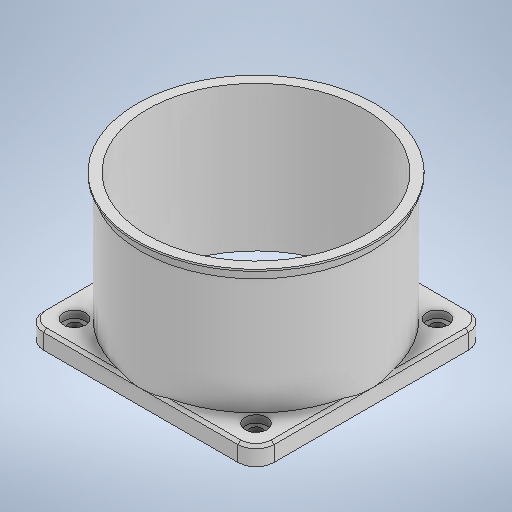
# Autodesk Inventor part: fanHoseMount
Saved by Autodesk Inventor 2025.1 (Build 291241000, 241)
## iProperties
Created: 2024-09-02
Part Number: fanHoseMount
Material: Generic
Document SubType Name: Modeling
Designer: Eric
Density: 1 g/cm^3
Appearance: Default
Author: Eric
Autodesk Inventor part; units mm, degrees
ref_plane "YZ Plane" through (0, 0, 0) normal (1, 0, 0) x (0, 1, 0)
ref_plane "XZ Plane" through (0, 0, 0) normal (0, 1, 0) x (-1, 0, 0)
ref_plane "XY Plane" through (0, 0, 0) normal (0, 0, 1) x (1, 0, 0)
sketch "Sketch1" plane through (0, 0, 0) normal (0, 1, 0) x (-1, 0, 0)
  circle A0 centre (0, 0) radius 30
  line L0 (26.75, -31.75) -> (-26.75, -31.75)
  line L1 (-31.75, -26.75) -> (-31.75, 26.75)
  line L2 (-26.75, 31.75) -> (26.75, 31.75)
  line L3 (31.75, 26.75) -> (31.75, -26.75)
  circle A1 centre (25, -25) radius 1.75
  circle A2 centre (-25, -25) radius 1.75
  circle A3 centre (-25, 25) radius 1.75
  circle A4 centre (25, 25) radius 1.75
  arc A5 (26.75, -31.75) -> (31.75, -26.75) centre (26.75, -26.75) ccw
  arc A6 (31.75, 26.75) -> (26.75, 31.75) centre (26.75, 26.75) ccw
  arc A7 (-26.75, 31.75) -> (-31.75, 26.75) centre (-26.75, 26.75) ccw
  arc A8 (-31.75, -26.75) -> (-26.75, -31.75) centre (-26.75, -26.75) ccw
  point P0 (31.75, -31.75)
  point P1 (0, -31.75)
  point P2 (-31.75, 0)
  dimension "d1" = 3.5
  dimension "d2" = 60
  dimension "d3" = 50
  dimension "d4" = 50
  dimension "d5" = 25
  dimension "d6" = 25
  dimension "d7" = 5
  dimension "d8" = 5
  dimension "d9" = 63.5
  dimension "d10" = 63.5
  constraints: 9 centre point, 8 end point, 8 point on circle, 8 tangent, 5 equal radius, 3 horizontal alignment, 3 vertical alignment, 2 midpoint, 2 parallel, 2 point on line, 1 coincident, 1 horizontal, 1 perpendicular
  measures "d1" diameter of A2
  measures "d2" diameter of A0
  measures "d3" distance of A1.centre A2.centre
  measures "d4" distance of A2.centre A3.centre
  measures "d5" horizontal distance of point (0, 0) A2.centre
  measures "d6" horizontal distance of point (0, 0) A2.centre
  measures "d7" radius of A5
  measures "d8" radius of A6
  measures "d9" distance between parallel lines of L2 L0
  measures "d10" distance between parallel lines of L3 L1
extrude "Extrusion1" add sketch "Sketch1" along normal blind 5
sketch "Sketch2" plane through (0, 5, 0) normal (0, 1, 0) x (1, 0, 0)
  circle A0 centre (-25, -25) radius 1.75 projected
  circle A1 centre (-25, -25) radius 3
  circle A2 centre (-25, 25) radius 1.75 projected
  circle A3 centre (-25, 25) radius 3
  circle A4 centre (25, 25) radius 1.75 projected
  circle A5 centre (25, 25) radius 3
  circle A6 centre (25, -25) radius 1.75 projected
  circle A7 centre (25, -25) radius 3
  point P0 (0, 0)
  dimension "d13" = 6
  constraints: 4 centre point, 4 coincident, 3 equal radius
  measures "d13" diameter of A1
extrude "Extrusion2" cut sketch "Sketch2" against normal blind 2 contours A0 | A1 | A2 | A3 | A4 | A5 | A6 | A7
sketch "Sketch3" plane through (0, 0, 0) normal (0, 0, 1) x (1, 0, 0)
  line L0 (-26.75, 5) -> (26.75, 5) projected
  line L1 (0, 5) -> (0, 15)
  arc A0 (0, 15) -> (0, 15) centre (30, 15) ccw
  line L2 (0, 15) -> (0, 40)
  point P0 (0, 0)
  dimension "d16" = 180
  dimension "d17" = 30
  dimension "d18" = 25
  dimension "d19" = 10
  constraints: 4 end point, 2 point on circle, 2 tangent, 1 centre point, 1 midpoint, 1 vertical
  measures "d16" angle of L1 L2
  measures "d17" radius of A0
  measures "d18" distance of L2.start L2.end
  measures "d19" distance of L1.start L1.end
sketch "Sketch4" plane through (0, 5, 0) normal (0, 1, 0) x (1, 0, 0)
  circle A0 centre (0, 0) radius 31.75
  line L0 (26.75, 31.75) -> (-26.75, 31.75) projected
  circle A1 centre (0, 0) radius 30 projected
  constraints: 1 centre point, 1 coincident, 1 tangent
sweep "Sweep1" add profiles "Sketch4" path "Sketch3" path curves L1 L2
sketch "Sketch5" plane through (0, 40, 0) normal (0, 1, 0) x (0, 0, -1)
  circle A0 centre (0, 0) radius 31.75 projected
  circle A1 centre (0, 0) radius 32.75
  point P0 (0, 0)
  dimension "d22" = 1
  constraints: 1 centre point
  measures "d22" radial gap between concentric circles of A0 A1
extrude "Extrusion3" add sketch "Sketch5" against normal blind 3
chamfer "Chamfer1" distance 1 distance2 2.5 1 edges at (0, 37, 32.75) measured on face at (0, 37, 32.25)
chamfer "Chamfer2" distance 0.75 angle 45 12 edges at (-31.75, 5, -13.375) (-30.2855, 5, -30.2855) (-13.375, 5, -31.75) (-31.75, 5, 13.375) (-30.2855, 5, 30.2855) (-13.375, 5, 31.75) (13.375, 5, -31.75) (30.2855, 5, -30.2855) (31.75, 5, -13.375) (13.375, 5, 31.75) (30.2855, 5, 30.2855) (31.75, 5, 13.375)
body "Solid1"
